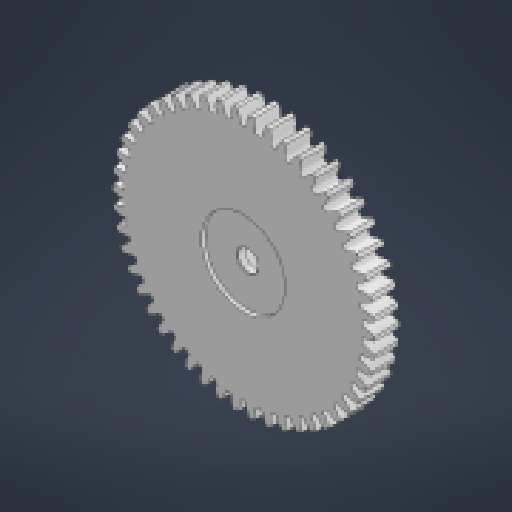
# Autodesk Inventor part: Bio50t
Saved by Autodesk Inventor 2024.1 (Build 281209000, 209)
## iProperties
Created: 2023-11-14
Part Number: Bio50t
Material: Generic
Document SubType Name: Modeling
Designer: Brandon
Density: 1 g/cm^3
Appearance: Default
Author: Brandon
Autodesk Inventor part; units mm, degrees
ref_plane "YZ Plane" through (0, 0, 0) normal (1, 0, 0) x (0, 1, 0)
ref_plane "XZ Plane" through (0, 0, 0) normal (0, 1, 0) x (-1, 0, 0)
ref_plane "XY Plane" through (0, 0, 0) normal (0, 0, 1) x (1, 0, 0)
sketch "Sketch1" plane through (0, 0, 0) normal (0, 0, 1) x (1, 0, 0)
  spline S0 degree 3 poles (-0.9188, 19.7907) (-0.8815, 19.705) (-0.8256, 19.5764) (-0.7585, 19.4019) (-0.711, 19.27) (-0.6668, 19.137) (-0.6263, 19.0028) (-0.5898, 18.8674) (-0.5582, 18.7308) (-0.5313, 18.5932) (-0.5187, 18.477) (-0.5079, 18.3842) (-0.4961, 18.315) (-0.479, 18.247) (-0.4568, 18.1804) (-0.4313, 18.1277) (-0.4066, 18.088) (-0.3855, 18.06) (-0.362, 18.034) (-0.3357, 18.0106) (-0.3067, 17.9909) (-0.2765, 17.973) (-0.2437, 17.9605) (-0.2101, 17.9504) (-0.1752, 17.9455) (-0.1051, 17.944) (0, 17.9464) (0.1051, 17.944) (0.1752, 17.9455) (0.2101, 17.9504) (0.2437, 17.9605) (0.2765, 17.973) (0.3067, 17.9909) (0.3357, 18.0106) (0.362, 18.034) (0.3855, 18.06) (0.4066, 18.088) (0.4313, 18.1277) (0.4568, 18.1804) (0.479, 18.247) (0.4961, 18.315) (0.5079, 18.3842) (0.5187, 18.477) (0.5313, 18.5932) (0.5582, 18.7308) (0.5898, 18.8674) (0.6263, 19.0028) (0.6668, 19.137) (0.711, 19.27) (0.7585, 19.4019) (0.8256, 19.5764) (0.8815, 19.705) (0.9188, 19.7907) knots 0 0 0 0 0.028034 0.042052 0.05607 0.070087 0.084105 0.098123 0.11214 0.126157 0.140172 0.14718 0.154188 0.161195 0.168201 0.175205 0.178708 0.18221 0.185714 0.189219 0.192721 0.196224 0.199727 0.20323 0.206733 0.210237 0.224255 0.238273 0.241778 0.24528 0.248784 0.252287 0.25579 0.259292 0.262797 0.266301 0.269803 0.273306 0.28031 0.287316 0.294323 0.301331 0.308339 0.322354 0.336371 0.350388 0.364406 0.378423 0.392441 0.406459 0.420477 0.448511 0.448511 0.448511 0.448511
  circle A0 centre (0, 0) radius 17.9453 construction
  circle A1 centre (0, 0) radius 18.4432 construction
  circle A2 centre (0, 0) radius 19.05 construction
  circle A3 centre (0, 0) radius 19.812
  point P0 (-0.8095, 19.5325)
  point P1 (-0.759, 19.4018)
  point P2 (-0.7116, 19.2698)
  point P3 (-0.6674, 19.1368)
  point P4 (-0.627, 19.0026)
  point P5 (-0.5906, 18.8672)
  point P6 (-0.559, 18.7307)
  point P7 (-0.5333, 18.5929)
  point P8 (-0.516, 18.4538)
  point P9 (-0.5073, 18.3842)
  point P10 (-0.4952, 18.3152)
  point P11 (-0.4781, 18.2472)
  point P12 (-0.4554, 18.181)
  point P13 (-0.4248, 18.118)
  point P14 (-0.4062, 18.0883)
  point P15 (-0.3851, 18.0604)
  point P16 (-0.3615, 18.0344)
  point P17 (-0.3352, 18.0112)
  point P18 (-0.3065, 17.9912)
  point P19 (-0.2761, 17.9739)
  point P20 (-0.2435, 17.9609)
  point P21 (-0.2099, 17.9513)
  point P22 (-0.1752, 17.9462)
  point P23 (-0.1402, 17.9448)
  point P24 (0, 17.9453)
  point P25 (0.1402, 17.9448)
  point P26 (0.1752, 17.9462)
  point P27 (0.2099, 17.9513)
  point P28 (0.2435, 17.9609)
  point P29 (0.2761, 17.9739)
  point P30 (0.3065, 17.9912)
  point P31 (0.3352, 18.0112)
  point P32 (0.3615, 18.0344)
  point P33 (0.3851, 18.0604)
  point P34 (0.4062, 18.0883)
  point P35 (0.4248, 18.118)
  point P36 (0.4554, 18.181)
  point P37 (0.4781, 18.2472)
  point P38 (0.4952, 18.3152)
  point P39 (0.5073, 18.3842)
  point P40 (0.516, 18.4538)
  point P41 (0.5333, 18.5929)
  point P42 (0.559, 18.7307)
  point P43 (0.5906, 18.8672)
  point P44 (0.627, 19.0026)
  point P45 (0.6674, 19.1368)
  point P46 (0.7116, 19.2698)
  point P47 (0.759, 19.4018)
  point P48 (0.8095, 19.5325)
  constraints: 4 centre point, 2 point on circle, 107 other
extrude "Extrusion1" add sketch "Sketch1" against normal blind 3.81
extrude "Extrusion2" cut sketch "Sketch1" against normal through all contours A3 S0 picked at (-0.0812, 19.1241)
pattern_circular "Circular Pattern1" count 50 over 360 about axis through (0, 0, 0) along (0, 0, -1) of "Extrusion2"
sketch "Sketch2" plane through (0, 0, -3.81) normal (0, 0, -1) x (-1, 0, 0)
  circle A0 centre (0, 0) radius 2.6
  circle A1 centre (0, 0) radius 1.55
  dimension "d7" = 5.2
  dimension "d8" = 3.1
  constraints: 2 centre point, 2 coincident
  measures "d7" diameter of A0
  measures "d8" diameter of A1
extrude "Extrusion3" cut sketch "Sketch2" against normal blind 2 contours A0 | A1
extrude "Extrusion4" cut sketch "Sketch2" against normal through all contours A1
sketch "Sketch3" plane through (0, 0, 0) normal (0, 0, 1) x (1, 0, 0)
  circle A0 centre (0, 0) radius 2.6 projected
  circle A1 centre (0, 0) radius 6.35
  dimension "d13" = 12.7
  constraints: 1 centre point, 1 coincident
  measures "d13" diameter of A1
extrude "Extrusion5" cut sketch "Sketch3" against normal blind 0.635 contours A0 | A1
chamfer "Chamfer1" distance 0.127 angle 45 2 edges at (1.55, 0, -0.635) (2.6, 0, -3.81)
equation "\"d0\" = FaceWidth"
equation "\"Module\" = 0.762"
equation "\"PressureAngle\" = 14.5deg"
equation "\"UnitProfileClearance\" = 0.25"
equation "\"UnitRoundRadius\" = 0.3335"
equation "\"HeadDiameter\" = 39.624"
equation "\"RootDiameter\" = 35.89066"
equation "\"BaseDiameter\" = 36.88643"
equation "\"PitchDiameter\" = 38.1"
equation "\"FaceWidth\" = 3.81"
equation "\"HelixAngle\" = 0"
equation "\"UnitCorrection\" = 0"
equation "\"UnitAddendumModification\" = 0"
equation "\"CircularPitch\" = 2.39389"
equation "\"UnitBacklashShift\" = -0.199696"
equation "\"TotalToolShift\" = -0.15217"
equation "\"IsInternal\" = 0"
body "Solid1"
